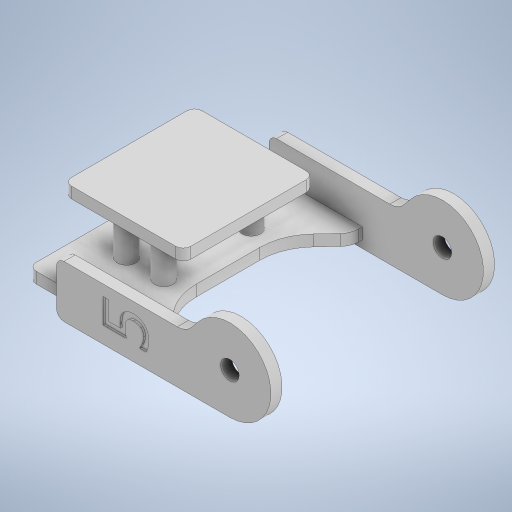
# Autodesk Inventor part: Pieza_5
Saved by Autodesk Inventor 2023 (Build 270158000, 158)
## iProperties
Created: 2024-09-27
Part Number: Pieza_5
Material: Genérico
Document SubType Name: Sheet Metal
Designer: sebas
Density: 1 g/cm^3
Sheet Metal Rule: Por defecto_mm
Appearance: Valor por defecto
Author: sebas
Autodesk Inventor part; units mm, degrees
ref_plane "Plano de trabajo1" through (0, 0, 27) normal (0, 0, 1) x (1, 0, 0)
sketch "Boceto1" plane through (0, 0, 27) normal (0, 0, 1) x (1, 0, 0)
  arc A0 (0, -11) -> (-8.5797, 6.8839) centre (0, 0) ccw
  line L0 (0, -11) -> (-44.5, -11)
  line L1 (-46.5, -9) -> (-46.5, 1)
  line L2 (-44.5, 3) -> (-14.0947, 3)
  line L3 (-10.1948, 4.8709) -> (-8.5797, 6.8839)
  arc A1 (-14.0947, 3) -> (-10.1948, 4.8709) centre (-14.0947, 8) ccw
  arc A2 (-44.5, 3) -> (-46.5, 1) centre (-44.5, 1) ccw
  arc A3 (-46.5, -9) -> (-44.5, -11) centre (-44.5, -9) ccw
  circle A4 centre (0, 0) radius 2.5
  point P0 (-46.5, -11)
  point P1 (-46.5, 3)
  point P2 (11, 0)
  dimension "d1" = 22
  dimension "d3" = 5
  dimension "d4" = 14
  dimension "d5" = 57.5
  dimension "d6" = 2
  dimension "d7" = 5
  constraints: 9 point on circle, 8 end point, 8 tangent, 5 centre point, 4 point on line, 2 coincident, 2 perpendicular, 1 equal radius, 1 horizontal
  measures "d1" diameter of A0
  measures "d3" radius of A1
  measures "d4" distance of point (-46.5, -11) point (-46.5, 3)
  measures "d5" distance from line of L1 point (11, 0)
  measures "d6" radius of A2
  measures "d7" diameter of A4
extrude "Extrusión1" add sketch "Boceto1" along normal blind 3
mirror "Simetría1" about plane through (0, 0, 0) normal (0, 0, 1) of "Extrusión1"
ref_plane "Plano de trabajo2" through (-44.5, -6, 27) normal (0, -1, 0) x (1, 0, 0)
sketch "Boceto2" plane through (-44.5, -6, 27) normal (0, -1, 0) x (1, 0, 0)
  line L0 (0, 0) -> (44.5, 0) projected
  line L1 (23, 0) -> (-10.5, 0)
  line L2 (-12.5, -2) -> (-12.5, -52)
  line L3 (-10.5, -54) -> (23, -54)
  line L4 (0, -54) -> (44.5, -54) projected
  line L5 (21.6267, -49.5581) -> (14, -41.5219)
  line L6 (14, -41.5219) -> (14, -12.4781)
  line L7 (14, -12.4781) -> (21.6267, -4.4419)
  line L8 (23, -1) -> (23, 0)
  line L9 (23, -53) -> (23, -54)
  line L10 (0, 3) -> (-2, 3) projected
  line L11 (14, -27) -> (-19.9317, -27) construction
  arc A0 (21.6267, -4.4419) -> (23, -1) centre (18, -1) ccw
  arc A1 (23, -53) -> (21.6267, -49.5581) centre (18, -53) ccw
  arc A2 (-10.5, 0) -> (-12.5, -2) centre (-10.5, -2) ccw
  arc A3 (-12.5, -52) -> (-10.5, -54) centre (-10.5, -52) ccw
  point P0 (44.5, -27)
  point P1 (-12.5, 0)
  point P2 (-12.5, -54)
  point P3 (-1, 3)
  dimension "d11" = 26.5
  dimension "d12" = 11.5
  dimension "d13" = 9
  dimension "d14" = 9
  dimension "d16" = 5
  dimension "d17" = 1
  dimension "d18" = 1
  dimension "d19" = 27
  dimension "d40" = 2
  constraints: 18 end point, 8 point on circle, 8 tangent, 6 point on line, 4 centre point, 2 collinear, 2 equal radius, 2 midpoint, 2 perpendicular, 1 horizontal, 1 parallel, 1 symmetric about line
  measures "d11" distance from line of L11.start L2
  measures "d12" distance from line of point (-1, 3) L2
  measures "d13" distance between parallel lines of L6 L9
  measures "d14" distance between parallel lines of L6 L8
  measures "d16" radius of A0
  measures "d17" distance of L8.start L1.start
  measures "d18" distance of L9.start L3.end
  measures "d19" distance between parallel lines of L0 L11
  measures "d40" radius of A2
extrude "Extrusión2" add sketch "Boceto2" along normal blind 3
ref_plane "Plano de trabajo3" through (-44.5, 6, 27) normal (0, 1, 0) x (1, 0, 0)
sketch "Boceto3" plane through (-44.5, 6, 27) normal (0, 1, 0) x (1, 0, 0)
  line L0 (-10.5, 44.5) -> (17.5, 44.5)
  line L1 (19.5, 42.5) -> (19.5, 11.5)
  line L2 (17.5, 9.5) -> (-10.5, 9.5)
  line L3 (-12.5, 11.5) -> (-12.5, 42.5)
  line L4 (0, 27) -> (-59, 27) construction
  line L5 (30.4053, 0) -> (0, 0) projected
  arc A0 (-10.5, 44.5) -> (-12.5, 42.5) centre (-10.5, 42.5) ccw
  arc A1 (-12.5, 11.5) -> (-10.5, 9.5) centre (-10.5, 11.5) ccw
  arc A2 (17.5, 9.5) -> (19.5, 11.5) centre (17.5, 11.5) ccw
  arc A3 (19.5, 42.5) -> (17.5, 44.5) centre (17.5, 42.5) ccw
  line L6 (-12.5, 2) -> (-12.5, 52) construction
  point P0 (44.5, 27)
  point P1 (-12.5, 44.5)
  point P2 (19.5, 44.5)
  point P3 (-12.5, 9.5)
  point P4 (-12.5, 27)
  point P5 (-12.5, 0)
  point P6 (-12.5, 54)
  dimension "d23" = 35
  dimension "d24" = 32
  dimension "d25" = 27
  dimension "d26" = 2
  constraints: 10 end point, 8 point on circle, 8 tangent, 6 point on line, 4 centre point, 3 equal radius, 2 horizontal, 2 midpoint, 2 parallel, 1 perpendicular, 1 other
  measures "d23" distance of point (-12.5, 9.5) point (-12.5, 44.5)
  measures "d24" distance of point (-12.5, 44.5) point (19.5, 44.5)
  measures "d25" distance between parallel lines of L5 L4
  measures "d26" radius of A0
extrude "Extrusión3" add sketch "Boceto3" along normal blind 3
sketch "Boceto4" plane through (-44.5, 9, 27) normal (0, 1, 0) x (1, 0, 0)
  line L0 (-12.5, 42.5) -> (-12.5, 11.5) construction
  line L1 (-12.5, 27) -> (20, 27) construction
  circle A0 centre (8.5, 38.75) radius 2.5
  circle A1 centre (-1.5, 38.75) radius 2.5
  line L2 (3.5, 27) -> (3.5, -23) construction
  circle A2 centre (8.5, 15.25) radius 2.5
  circle A3 centre (-1.5, 15.25) radius 2.5
  point P0 (44.5, 27)
  dimension "d29" = 5
  dimension "d30" = 10
  dimension "d31" = 16
  dimension "d32" = 11.75
  constraints: 4 centre point, 4 end point, 3 symmetric about line, 1 horizontal, 1 midpoint, 1 point on line, 1 vertical, 2 other
  measures "d29" diameter of A1
  measures "d30" distance of A1.centre A0.centre
  measures "d31" distance between parallel lines of L2 L0
  measures "d32" distance from line of A0.centre L1
extrude "Extrusión4" cut sketch "Boceto4" against normal up to surface (18 mm away)
fillet "Empalme1" radius 15 2 edges at (-30.5, -7.5, 14.5219) (-30.5, -7.5, -14.5219)
sketch "Boceto5" plane through (0, 0, 30) normal (0, 0, 1) x (1, 0, 0)
  line L0 (-34, -8) -> (-34, 17.5513) construction
  line L1 (-34, 17.5513) -> (-23.3891, 17.5513) construction
  line L2 (-23.3891, 17.5513) -> (-23.3891, -8) construction
  line L3 (-23.3891, -8) -> (-34, -8) construction
  spline S0 degree 2 poles (-25.812, 0.1491) (-24.9465, 0.1491) (-23.4684, -0.4052) (-22.9238, -0.9109) knots 0 0 0 1 2 2 2
  spline S1 degree 2 poles (-22.9238, -0.9109) (-22.3793, -1.4165) (-21.7472, -2.9238) (-21.7472, -3.8574) knots 0 0 0 1 2 2 2
  spline S2 degree 2 poles (-21.7472, -3.8574) (-21.7472, -4.7131) (-22.1264, -6.3857) (-22.4279, -6.9984) knots 0 0 0 1 2 2 2
  line L4 (-22.4279, -6.9984) -> (-24.1297, -6.9984)
  line L5 (-24.1297, -6.9984) -> (-24.1297, -6.8817)
  spline S3 degree 2 poles (-24.1297, -6.8817) (-23.9935, -6.6969) (-23.6434, -6.0065) (-23.4878, -5.5883) knots 0 0 0 1 2 2 2
  spline S4 degree 2 poles (-23.4878, -5.5883) (-23.3225, -5.1118) (-23.1378, -4.3241) (-23.1378, -3.8282) knots 0 0 0 1 2 2 2
  spline S5 degree 2 poles (-23.1378, -3.8282) (-23.1378, -3.342) (-23.4878, -2.4279) (-23.8671, -2.0972) knots 0 0 0 1 2 2 2
  spline S6 degree 2 poles (-23.8671, -2.0972) (-24.2269, -1.7958) (-25.1799, -1.4846) (-25.8217, -1.4846) knots 0 0 0 1 2 2 2
  spline S7 degree 2 poles (-25.8217, -1.4846) (-26.4635, -1.4846) (-27.2804, -1.8347) (-27.5527, -2.1653) knots 0 0 0 1 2 2 2
  spline S8 degree 2 poles (-27.5527, -2.1653) (-27.8541, -2.5057) (-28.107, -3.517) (-28.107, -4.1297) knots 0 0 0 1 2 2 2
  spline S9 degree 2 poles (-28.107, -4.1297) (-28.107, -4.7909) (-27.9028, -6.1037) (-27.8152, -6.5024) knots 0 0 0 1 2 2 2
  line L6 (-27.8152, -6.5024) -> (-34, -6.5024)
  line L7 (-34, -6.5024) -> (-34, 0.081)
  line L8 (-34, 0.081) -> (-32.59, 0.081)
  line L9 (-32.59, 0.081) -> (-32.59, -4.9562)
  line L10 (-32.59, -4.9562) -> (-29.3906, -4.9562)
  spline S10 degree 2 poles (-29.3906, -4.9562) (-29.4295, -4.6645) (-29.4587, -4.1005) (-29.4587, -3.8671) knots 0 0 0 1 2 2 2
  spline S11 degree 2 poles (-29.4587, -3.8671) (-29.4587, -2.9433) (-29.1572, -1.6694) (-28.7099, -1.0859) knots 0 0 0 1 2 2 2
  spline S12 degree 2 poles (-28.7099, -1.0859) (-28.2626, -0.4927) (-26.9011, 0.1491) (-25.812, 0.1491) knots 0 0 0 1 2 2 2
  point P0 (0, 0)
  constraints: 2 other
extrude "Extrusión5" cut sketch "Boceto5" against normal blind 0.5
ref_plane "Plano de trabajo4" through (-44.5, 0, 27) normal (0, -1, 0) x (1, 0, 0)
sketch "Boceto6" plane through (-44.5, 0, 27) normal (0, -1, 0) x (1, 0, 0)
  circle A0 centre (8.5, -15.25) radius 2.5 projected
  circle A1 centre (-1.5, -15.25) radius 2.5 projected
  circle A2 centre (8.5, -38.75) radius 2.5 projected
  circle A3 centre (-1.5, -38.75) radius 2.5 projected
  point P0 (44.5, -27)
extrude "Extrusión6" add sketch "Boceto6" along normal mid plane 18
equation "\"Radio_pliegue\" = Grosor"
equation "\"Anchura_desahogo_plegado\" = Grosor"
equation "\"Profundidad_desahogo_plegado\" = 0.5 * Grosor"
equation "\"Tamaño_destalonado\" = 4 * Grosor"
equation "\"Remanente_mínimo\" = 2 * Grosor"
equation "\"Radiodetransición\" = Radio_pliegue"
equation "\"Tamaño_de_radio_de_Jacobi\" = Radio_pliegue"
equation "\"TamañoSeparación\" = Grosor"
equation "\"Grosor\" = 0.5"
